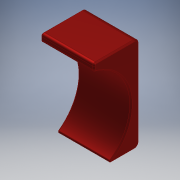
# Autodesk Inventor part: EPS_BatteryHeatsink
Saved by Autodesk Inventor 2018 (Build 220112000, 112)
## iProperties
Created: 2018-09-29
Part Number: EPS_BatteryHeatsink
Material: Aluminum 6061
Document SubType Name: Modeling
Designer: Bradley
Density: 2.7 g/cm^3
Appearance: Anodized - Red
Mass: 4.62891 g
Surface Area: 16.2557 cm^2
Volume: 1.71441 cm^3
Author: Bradley
Autodesk Inventor part; units mm, degrees
ref_plane "YZ Plane" through (0, 0, 0) normal (1, 0, 0) x (0, 1, 0)
ref_plane "XZ Plane" through (0, 0, 0) normal (0, 1, 0) x (-1, 0, 0)
ref_plane "XY Plane" through (0, 0, 0) normal (0, 0, 1) x (1, 0, 0)
sketch "Sketch1" plane through (0, 0, 0) normal (1, 0, 0) x (0, 1, 0)
  line L0 (4.45, 9.25) -> (4.45, -9.25)
  line L1 (4.45, -9.25) -> (-1.8065, -9.25)
  arc A0 (-1.8065, -9.25) -> (-4.45, 7.7812) centre (-6.45, -1.25) ccw
  line L2 (4.45, 9.25) -> (-4.45, 9.25)
  circle A1 centre (-6.45, -1.25) radius 9.15 construction
  line L3 (4.45, 6.063) -> (-0.7859, 6.063) construction
  line L4 (-4.45, 9.25) -> (-4.45, 7.7812)
  point P0 (0, 0)
  point P1 (0, 9.25)
  point P2 (4.45, 0)
  dimension "d0" = 10.9
  dimension "d1" = 18.3
  dimension "d2" = 0.1
  dimension "d6" = 8
  dimension "d7" = 7.313
  dimension "d9" = 2
  dimension "d19" = 10.5
  constraints: 10 end point, 3 point on circle, 2 centre point, 2 horizontal, 2 midpoint, 1 coincident, 1 horizontal alignment, 1 parallel, 1 perpendicular, 1 point on line, 1 vertical, 1 vertical alignment
  measures "d0" distance from line of A0.centre L0
  measures "d1" diameter of A1
  measures "d2" radial gap between concentric circles of A1 A0
  measures "d6" distance from line of L1 A0.centre
  measures "d7" distance from line of L3 A0.centre
  measures "d9" distance from line of A0.centre L4
  measures "d19" distance from line of A0.centre L2
extrude "Extrusion1" add sketch "Sketch1" along normal mid plane 10.4
sketch "Sketch2" plane through (-5.2, 4.45, 9.25) normal (0, 1, 0) x (1, 0, 0)
  line L0 (0, 0) -> (10.4, 0) projected
  line L1 (10.4, 18.5) -> (10.4, 0) projected
  line L2 (10.4, 18.5) -> (0, 18.5) projected
  line L3 (0, 0) -> (0, 18.5) projected
  line L4 (0, 0) -> (10.4, 0) construction
  line L5 (5.2, 0) -> (5.2, 18.5) construction
  line L6 (10.4, 18.5) -> (0, 18.5) construction
  point P0 (5.2, 9.25)
  point P1 (5.2, 3.187)
  point P2 (5.2, 3.187)
  point P3 (5.2, 3.187)
  point P4 (5.2, 3.187)
  constraints: 2 end point, 2 midpoint, 1 symmetric about line
hole "Hole1" at (0, 4.45, 6.063) at (0, 4.45, 6.063) direction (0, -1, 0) diameter 2.459 end through all thread size "M3x0.5" class "6H" standard "ANSI Metric M Profile"
fillet "Fillet1" radius 1 2 edges at (0, 4.45, 9.25) (0, 4.45, -9.25)
fillet "Fillet1" radius 0.5 2 edges at (0, -4.45, 9.25) (0, -4.45, 7.7812)
fillet "Fillet1" radius 0.25 1 edges at (0, -1.8065, -9.25)
chamfer "Chamfer1" distance 0.25 angle 45 20 edges at (5.2, -0.25, 9.25) (5.2, -4.3036, 9.1036) (5.2, -4.45, 8.462) (5.2, -4.3463, 7.8692) (5.2, 2.6527, 0.3942) (5.2, -1.1939, -9.0759) (5.2, 1.2472, -9.25) (5.2, 4.1571, -8.9571) (5.2, 4.45, 0) (5.2, 4.1571, 8.9571) (-5.2, -0.25, 9.25) (-5.2, 4.1571, 8.9571) (-5.2, 4.45, 0) (-5.2, 4.1571, -8.9571) (-5.2, 1.2472, -9.25) (-5.2, -1.1939, -9.0759) (-5.2, 2.6527, 0.3942) (-5.2, -4.3463, 7.8692) (-5.2, -4.45, 8.462) (-5.2, -4.3036, 9.1036)
body "Solid1"
